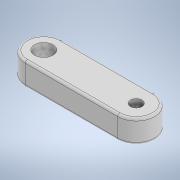
# Autodesk Inventor part: G-5
Saved by Autodesk Inventor 2021 (Build 250183000, 183)
## iProperties
Created: 2021-06-28
Part Number: G-5
Material: Generic
Document SubType Name: Modeling
Designer: Ranjita
Density: 1 g/cm^3
Appearance: Default
Author: Ranjita
Autodesk Inventor part; units mm, degrees
ref_plane "YZ Plane" through (0, 0, 0) normal (1, 0, 0) x (0, 1, 0)
ref_plane "XZ Plane" through (0, 0, 0) normal (0, 1, 0) x (-1, 0, 0)
ref_plane "XY Plane" through (0, 0, 0) normal (0, 0, 1) x (1, 0, 0)
sketch "Sketch1" plane through (0, 0, 0) normal (0, 1, 0) x (-1, 0, 0)
  line L0 (0, 0) -> (-13.33, 0) construction
  line L1 (0, -2.665) -> (-13.33, -2.665)
  line L2 (-13.33, 2.665) -> (0, 2.665)
  arc A0 (0, -2.665) -> (0, 2.665) centre (0, 0) ccw
  arc A1 (-13.33, 2.665) -> (-13.33, -2.665) centre (-13.33, 0) ccw
  circle A2 centre (-13.33, 0) radius 0.83
  circle A3 centre (0, 0) radius 1.33
  point P0 (-6.665, 0)
  dimension "d0" = 5.33
  dimension "d1" = 13.33
  dimension "d2" = 2.66
  dimension "d3" = 1.66
  constraints: 8 end point, 4 centre point, 4 point on circle, 4 tangent, 2 coincident, 1 horizontal, 1 midpoint, 1 parallel
  measures "d0" distance between parallel lines of L1 L2
  measures "d1" distance of L2.start L2.end
  measures "d2" diameter of A3
  measures "d3" diameter of A2
extrude "Extrusion1" add sketch "Sketch1" along normal blind 3.33
fillet "Fillet1" radius 0.33 8 edges at (6.665, 0, -2.665) (6.665, 3.33, -2.665) (-2.665, 0, 0) (6.665, 0, 2.665) (15.995, 0, 0) (-2.665, 3.33, 0) (6.665, 3.33, 2.665) (15.995, 3.33, 0)
body "Solid1"
